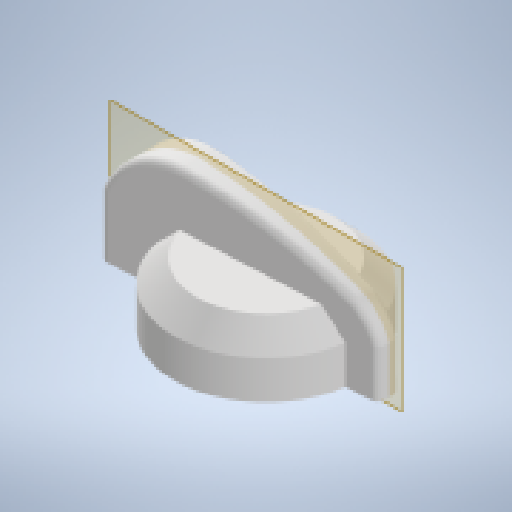
# Autodesk Inventor part: knob_holder
Saved by Autodesk Inventor 2023.1 (Build 271208000, 208)
## iProperties
Created: 2022-12-24
Part Number: knob_holder
Material: Generic
Document SubType Name: Modeling
Designer: USER
Density: 1 g/cm^3
Appearance: Default
Author: USER
Autodesk Inventor part; units mm, degrees
ref_plane "YZ Plane" through (0, 0, 0) normal (1, 0, 0) x (0, 1, 0)
ref_plane "XZ Plane" through (0, 0, 0) normal (0, 1, 0) x (-1, 0, 0)
ref_plane "XY Plane" through (0, 0, 0) normal (0, 0, 1) x (1, 0, 0)
sketch "Sketch1" plane through (0, 0, 0) normal (0, 1, 0) x (-1, 0, 0)
  circle A0 centre (0, 0) radius 26.5
  circle A1 centre (0, 0) radius 20
  line L0 (41, 6.787877) -> (41, -6.712123)
  line L1 (-35.2, 2.946468) -> (-35.2, -3.253532)
  line L2 (41, 6.787877) -> (-35.2, 2.946468)
  line L3 (41, -6.712123) -> (-35.2, -3.253532)
  dimension "d0" = 53
  dimension "d1" = 40
  dimension "d4" = 13.5
  dimension "d5" = 6.2
  dimension "d6" = 14.5
  dimension "d7" = 8.7
  constraints: 8 end point, 2 centre point, 2 coincident, 2 vertical
  measures "d0" diameter of A0
  measures "d1" diameter of A1
  measures "d4" distance of L0.start L0.end
  measures "d5" distance of L1.start L1.end
  measures "d6" distance edge to line of A0 L0
  measures "d7" distance edge to line of A0 L1
extrude "Extrusion1" add sketch "Sketch1" along normal blind 11 contours A0 L3 A1 L2 | L2 A1 A0 | A0 L3 A1 | L2 A1 L3 A0
extrude "Extrusion2" add sketch "Sketch1" along normal blind 17.5 contours L2 A1 | A1 L3 L2 | A1 L3
chamfer "Chamfer1" distance 6.5 angle 45 1 edges at (20, 11, 0)
extrude "Extrusion3" add sketch "Sketch1" along normal blind 32.7 contours A0 L3 A1 L2 | A0 L2 L0 L3 | L2 A1 L3 A0 | A0 L3 L1 L2 | A1 L3 L2
ref_plane "Work Plane1" through (99.917808, 0, -0.316099) normal (0.0025062, 0, 0.9999969) x (0, -1, 0)
sketch "Sketch2" plane through (99.917808, 0, -0.316099) normal (0.0025062, 0, 0.9999969) x (0, -1, 0)
  line L0 (-32.7, -140.935169) -> (-32.7, -64.725782)
  line L1 (0, -140.935169) -> (-32.7, -140.935169)
  arc A0 (-32.7, -119.250258) -> (-17.777908, -140.935169) centre (-8.821667, -118.795445) ccw
  arc A1 (-22.798943, -72.859474) -> (-32.7, -119.250258) centre (98.656685, -123.033384) ccw
  line L2 (0, -64.725782) -> (-32.7, -64.725782)
  arc A2 (-13.517437, -64.725782) -> (-22.798943, -72.859474) centre (-9.938612, -78.172139) ccw
  line L3 (-16.35, -140.935169) -> (-16.35, -146.892817)
  line L4 (-16.35, -146.892817) -> (-43.194783, -146.892817)
  line L5 (-43.194783, -146.892817) -> (-41.628509, -60.616947)
  line L6 (-41.628509, -60.616947) -> (-16.35, -59.453881)
  line L7 (-16.35, -59.453881) -> (-13.517437, -64.725782)
  point P0 (0, -99.918287)
  constraints: 10 end point, 6 point on circle, 4 point on line, 3 centre point, 1 midpoint, 1 perpendicular, 1 tangent, 1 vertical
extrude "Extrusion4" cut sketch "Sketch2" along normal mid plane 67.625
fillet "Fillet1" radius 2 10 edges at (-32.4, 28.4962, 6.3543) (32.2188, 19.1093, 3.0968) (4.3252, 29.86, 4.5029) (-41, 8.889, 6.7879) (-41, 8.9305, -6.7121) (-32.3948, 28.5216, -6.3215) (32.2025, 19.1093, -3.3896) (4.3022, 29.86, -4.6559) (35.2, 6.7587, 2.9465) (35.2, 6.7629, -3.2535)
body "Solid1"
